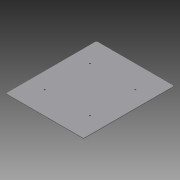
# Autodesk Inventor part: 000103
Saved by Autodesk Inventor 2015 (Build 190159000, 159)
## iProperties
Created: 2015-05-11
Part Number: 000103
Material: Generic
Document SubType Name: Modeling
Designer: Wesley
Density: 1 g/cm^3
Appearance: Default
Author: Wesley
Autodesk Inventor part; units mm, degrees
ref_plane "YZ Plane" through (0, 0, 0) normal (1, 0, 0) x (0, 1, 0)
ref_plane "XZ Plane" through (0, 0, 0) normal (0, 1, 0) x (-1, 0, 0)
ref_plane "XY Plane" through (0, 0, 0) normal (0, 0, 1) x (1, 0, 0)
sketch "Sketch1" plane through (0, 0, 0) normal (0, 1, 0) x (-1, 0, 0)
  line L0 (0, 0) -> (152.4, 0)
  line L1 (152.4, 0) -> (152.4, -177.8)
  line L2 (152.4, -177.8) -> (0, -177.8)
  line L3 (0, -177.8) -> (0, 0)
  dimension "d0" = 152.4
  dimension "d1" = 177.8
  constraints: 8 end point, 2 parallel, 1 horizontal, 1 perpendicular
  measures "d0" distance of L0.start L0.end
  measures "d1" distance of L2.end L0.start
extrude "Extrusion1" add sketch "Sketch1" along normal blind 1.27
sketch "Sketch2" plane through (0, 1.27, 0) normal (0, 1, 0) x (1, 0, 0)
  line L0 (0, 0) -> (-31.75, 0) construction
  line L1 (-31.75, 0) -> (-31.75, 44.45) construction
  line L2 (-31.75, 44.45) -> (0, 44.45) construction
  line L3 (0, 44.45) -> (0, 0) construction
  line L4 (-152.4, 0) -> (-120.65, 0) construction
  line L5 (-120.65, 0) -> (-120.65, 44.45) construction
  line L6 (-120.65, 44.45) -> (-152.4, 44.45) construction
  line L7 (-152.4, 44.45) -> (-152.4, 0) construction
  line L8 (-152.4, 177.8) -> (-120.65, 177.8) construction
  line L9 (-120.65, 177.8) -> (-120.65, 133.35) construction
  line L10 (-120.65, 133.35) -> (-152.4, 133.35) construction
  line L11 (-152.4, 133.35) -> (-152.4, 177.8) construction
  line L12 (0, 177.8) -> (-31.75, 177.8) construction
  line L13 (-31.75, 177.8) -> (-31.75, 133.35) construction
  line L14 (-31.75, 133.35) -> (0, 133.35) construction
  line L15 (0, 133.35) -> (0, 177.8) construction
  dimension "d4" = 44.45
  dimension "d5" = 31.75
  dimension "d6" = 31.75
  dimension "d7" = 44.45
  dimension "d8" = 44.45
  dimension "d9" = 31.75
  dimension "d10" = 44.45
  constraints: 32 end point, 8 parallel, 4 horizontal, 4 perpendicular, 1 point on line
  measures "d4" distance of L2.end L0.start
  measures "d5" distance of L0.start L0.end
  measures "d6" distance of L4.start L4.end
  measures "d7" distance of L6.end L4.start
  measures "d8" distance of L10.end L8.start
  measures "d9" distance of L12.start L12.end
  measures "d10" distance of L14.end L12.start
hole "Hole1" at (-152.4, 1.27, 0) at (-152.4, 1.27, -177.8) at (0, 1.27, -177.8) at (-120.65, 1.27, -133.35) at (-31.75, 1.27, -133.35) at (-31.75, 1.27, -44.45) at (-120.65, 1.27, -44.45) direction (0, -1, 0) diameter 3.1953 end through all
body "Solid1"
